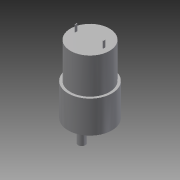
# Autodesk Inventor part: 37D
Saved by Autodesk Inventor 2015 (Build 190159000, 159)
## iProperties
Created: 2012-05-16
Part Number: 37D
Document SubType Name: Modeling
Designer: David
Density: 1 g/cm^3
Mass: 49.1572 g
Surface Area: 89.8245 cm^2
Volume: 49.1572 cm^3
Material: Genérico
Appearance: Acero
Author: David
Autodesk Inventor part; units mm, degrees
ref_plane "YZ Plane" through (0, 0, 0) normal (1, 0, 0) x (0, 1, 0)
ref_plane "XZ Plane" through (0, 0, 0) normal (0, 1, 0) x (-1, 0, 0)
ref_plane "XY Plane" through (0, 0, 0) normal (0, 0, 1) x (1, 0, 0)
sketch "Boceto1" plane through (0, 0, 0) normal (0, 0, 1) x (1, 0, 0)
  circle A0 centre (0, 0) radius 18.4
  dimension "d0" = 36.8
  constraints: 1 centre point
  measures "d0" diameter of A0
extrude "Extrusión1" add sketch "Boceto1" along normal blind 27
sketch "Boceto2" plane through (0, 0, 27) normal (0, 0, 1) x (1, 0, 0)
  circle A0 centre (0, 0) radius 18.4 projected
  circle A1 centre (0, 0) radius 16.4
  dimension "d4" = 2
  constraints: 1 centre point, 1 coincident
  measures "d4" radial gap between concentric circles of A0 A1
extrude "Extrusión2" add sketch "Boceto2" along normal blind 30 contours A1
sketch "Boceto3" plane through (0, 0, 57) normal (0, 0, 1) x (1, 0, 0)
  circle A0 centre (0, 0) radius 16.4 projected
  line L0 (0, 0) -> (12.05, 0)
  line L1 (0, 0) -> (-12.05, 0)
  line L2 (-12.05, 0) -> (-12.05, 1)
  line L3 (-12.05, 1) -> (-12, 1)
  line L4 (-12, 1) -> (-12, -1)
  line L5 (-12, -1) -> (-12.05, -1)
  line L6 (-12.05, -1) -> (-12.05, 0)
  line L7 (12.05, 0) -> (12.05, 1)
  line L8 (12.05, 1) -> (12, 1)
  line L9 (12, 1) -> (12, -1)
  line L10 (12, -1) -> (12.05, -1)
  line L11 (12.05, -1) -> (12.05, 0)
  dimension "d7" = 12.05
  dimension "d8" = 12.05
  constraints: 24 end point, 4 perpendicular, 3 collinear, 3 parallel, 1 horizontal, 1 point on line
  measures "d7" distance of L0.start L0.end
  measures "d8" distance of L0.start L1.end
extrude "Extrusión3" add sketch "Boceto3" along normal blind 5.6 contours L9 L8 L7 L0 | L0 L11 L10 L9 | L4 L5 L6 L1 | L1 L2 L3 L4
sketch "Boceto4" plane through (0, 0, 0) normal (0, 0, -1) x (-1, 0, 0)
  circle A0 centre (13.4234, -7.75) radius 1.5
  circle A1 centre (13.4234, 7.75) radius 1.5
  circle A2 centre (0, 15.5) radius 1.5
  circle A3 centre (-13.4234, 7.75) radius 1.5
  circle A4 centre (-13.4234, -7.75) radius 1.5
  circle A5 centre (0, -15.5) radius 1.5
  line L0 (0, 0) -> (7, 0)
  circle A6 centre (7, 0) radius 6
  arc A7 (7.2895, 7.9948) -> (7.2895, -7.9948) centre (7, 0) ccw
  arc A8 (7.9572, 9.7695) -> (7.9572, -9.7695) centre (0, 0) ccw
  arc A9 (7.9572, -9.7695) -> (7.2895, -7.9948) centre (7.3257, -8.9941) ccw
  arc A10 (7.2895, 7.9948) -> (7.9572, 9.7695) centre (7.3257, 8.9941) ccw
  dimension "d19" = 7
  dimension "d20" = 12
  dimension "d34" = 1
  constraints: 11 centre point, 8 point on circle, 4 tangent, 2 coincident, 2 end point, 1 equal radius
  measures "d19" distance of L0.start L0.end
  measures "d20" diameter of A6
  measures "d34" radius of A9
extrude "Extrusión4" add sketch "Boceto4" along normal blind 6 contours A6
sketch "Boceto5" plane through (-7, 0, -6) normal (0, 0, -1) x (-1, 0, 0)
  circle A0 centre (0, 0) radius 6 projected
  line L0 (6, 0) -> (0, 0)
  line L1 (0, 6) -> (0, 0)
  constraints: 4 end point, 2 point on circle
extrude "Extrusión5" add sketch "Boceto5" along normal blind 0.5 contours L0 L1 A0 picked at (3.9499, 0.445)
sketch "Boceto6" plane through (0, 0, -6) normal (0, 0, -1) x (-1, 0, 0)
  line L0 (13, 0) -> (7, 0) projected
  line L1 (7, 0) -> (7, 6) projected
  arc A0 (7, 6) -> (13, 0) centre (7, 0) ccw projected
extrude "Extrusión6" cut sketch "Boceto6" against normal blind 0.5
sketch "Boceto7" plane through (-7, 0, -6.5) normal (1, 0, 0) x (0, 0, -1)
  line L0 (0, 0) -> (0, 6) projected
  line L1 (-1, 0) -> (0, 0) projected
  line L2 (-1, 6) -> (0, 5)
  line L3 (0, 5) -> (0, 6)
  line L4 (-1, 6) -> (0, 5)
  line L5 (-1, 6) -> (0, 6)
  line L6 (-1, 6) -> (0, 5)
  line L7 (0, 5) -> (-1, 6)
  constraints: 12 end point, 3 collinear, 1 perpendicular
revolve "Revolución1" cut sketch "Boceto7" angle 360 about axis through (-7, 0, -5.5) along (0, 0, -1)
sketch "Boceto8" plane through (-7, 0, -5.5) normal (1, 0, 0) x (0, 0, -1)
  line L0 (1, 5) -> (0, 6) projected
  line L1 (0, 0) -> (0, 6) projected
  line L2 (0, 0) -> (1, 0) projected
  line L3 (1, 0) -> (1, 5) projected
revolve "Revolución2" add sketch "Boceto8" angle 360 about axis through (-7, 0, -5.5) along (0, 0, -1)
sketch "Boceto9" plane through (-7, 0, -6.5) normal (0, 0, -1) x (-1, 0, 0)
  circle A0 centre (0, 0) radius 5 projected
  circle A1 centre (0, 0) radius 3
  constraints: 1 centre point, 1 coincident
extrude "Extrusión7" add sketch "Boceto9" along normal blind 15.5 contours A1
sketch "Boceto10" plane through (-7, 0, -22) normal (0, 0, -1) x (-1, 0, 0)
  circle A0 centre (0, 0) radius 3 projected
  line L0 (1.6583, 2.5) -> (-1.6583, 2.5)
  constraints: 2 end point, 2 point on circle
extrude "Extrusión8" cut sketch "Boceto10" against normal blind 12 contours L0 A0 picked at (-0.1169, 2.6598)
extrude "Extrusión9" cut sketch "Boceto4" against normal blind 1 contours A7 A9 A8 A10
extrude "Extrusión10" cut sketch "Boceto4" against normal blind 10 contours A0 | A1 | A2 | A3 | A4 | A5
sketch "Boceto12" plane through (-12, -1, 57) normal (1, 0, 0) x (0, 0, -1)
  line L0 (-5.6, 2) -> (-5.6, 0) projected
  line L1 (0, 0) -> (-5.6, 0) projected
  line L2 (0, 2) -> (0, 0) projected
  line L3 (0, 2) -> (-5.6, 2) projected
extrude "Extrusión11" add sketch "Boceto12" along normal blind 0.45
sketch "Boceto13" plane through (12, -1, 57) normal (-1, 0, 0) x (0, 0, 1)
  line L0 (5.6, 0) -> (5.6, 2) projected
  line L1 (0, 2) -> (5.6, 2) projected
  line L2 (0, 0) -> (0, 2) projected
  line L3 (0, 0) -> (5.6, 0) projected
extrude "Extrusión12" add sketch "Boceto13" along normal blind 0.45
sketch "Boceto14" plane through (0, 0, 0) normal (0, 0, -1) x (-1, 0, 0)
  circle A0 centre (0, -15.5) radius 1.5 projected
  circle A1 centre (-13.4234, -7.75) radius 1.5 projected
  circle A2 centre (-13.4234, 7.75) radius 1.5 projected
  circle A3 centre (13.4234, 7.75) radius 1.5 projected
  circle A4 centre (13.4234, -7.75) radius 1.5 projected
  circle A5 centre (0, 15.5) radius 1.5 projected
  arc A6 (7.2895, 7.9948) -> (7.2895, -7.9948) centre (7, 0) ccw projected
  arc A7 (7.9572, -9.7695) -> (7.2895, -7.9948) centre (7.3257, -8.9941) ccw projected
  arc A8 (7.9572, 9.7695) -> (7.9572, -9.7695) centre (0, 0) ccw projected
  arc A9 (7.2895, 7.9948) -> (7.9572, 9.7695) centre (7.3257, 8.9941) ccw projected
  circle A10 centre (7, 0) radius 6 projected
  circle A11 centre (0, 0) radius 18.4 projected
sketch "Boceto15" plane through (-7, 0, -22) normal (0, 0, -1) x (-1, 0, 0)
  line L0 (1.6583, 2.5) -> (-1.6583, 2.5) projected
  arc A0 (-1.6583, 2.5) -> (1.6583, 2.5) centre (0, 0) ccw projected
